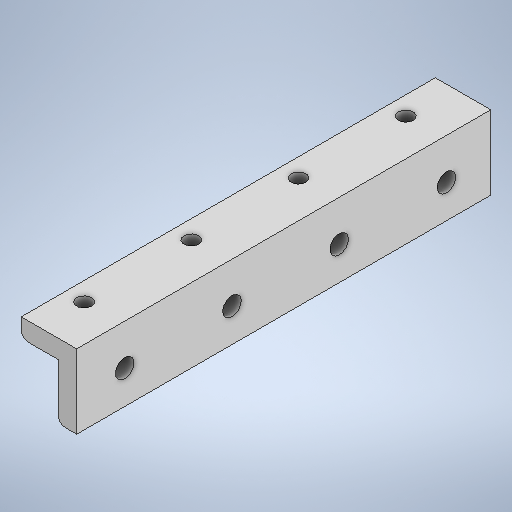
# Autodesk Inventor part: 1014
Saved by Autodesk Inventor 2025.1 (Build 291241000, 241)
## iProperties
Created: 2024-06-10
Part Number: 1014
Material: Generisch
Document SubType Name: Modeling
Designer: ffogue
Density: 1 g/cm^3
Appearance: Vorgabe
Author: ffogue
Autodesk Inventor part; units mm, degrees
ref_plane "YZ Plane" through (0, 0, 0) normal (1, 0, 0) x (0, 1, 0)
ref_plane "XZ Plane" through (0, 0, 0) normal (0, 1, 0) x (-1, 0, 0)
ref_plane "XY Plane" through (0, 0, 0) normal (0, 0, 1) x (1, 0, 0)
sketch "Skizze2" plane through (0, 0, 0) normal (0, 1, 0) x (-1, 0, 0)
  line L0 (0, 0) -> (15, 0)
  line L1 (15, 0) -> (15, -5)
  line L2 (15, -5) -> (5, -5)
  line L3 (5, -5) -> (5, -20)
  line L4 (5, -20) -> (0, -20)
  line L5 (0, -20) -> (0, 0)
  dimension "d6" = 5
  dimension "d7" = 15
  dimension "d8" = 5
  dimension "d9" = 10
  constraints: 12 end point, 5 perpendicular, 1 horizontal
  measures "d6" distance between parallel lines of L2 L0
  measures "d7" distance between parallel lines of L2 L4
  measures "d8" distance between parallel lines of L5 L3
  measures "d9" distance between parallel lines of L3 L1
extrude "Extrusion1" add sketch "Skizze2" along normal blind 112
sketch "Skizze3" plane through (-5, 0, -5) normal (0, 0, -1) x (-1, 0, 0)
  line L0 (0, 112) -> (10, 112) projected
  line L1 (-5, 0) -> (-5, 112) projected
  point P0 (5, 99)
  point P1 (5, 70)
  point P2 (5, 41)
  point P3 (5, 12)
  point P4 (5, 112)
  point P5 (5, 112)
  dimension "d12" = 13
  dimension "d13" = 29
  dimension "d14" = 29
  dimension "d15" = 29
  dimension "d39" = 10
  constraints: 4 vertical alignment, 2 midpoint
  measures "d12" distance of point (5, 112) point (5, 99)
  measures "d13" distance of point (5, 70) point (5, 99)
  measures "d14" distance of point (5, 41) point (5, 70)
  measures "d15" distance of point (5, 12) point (5, 41)
  measures "d39" distance from line of L1 point (5, 99)
hole "Bohrung1" at (-10, 99, -5) at (-10, 70, -5) at (-10, 41, -5) at (-10, 12, -5) direction (0, 0, 1) diameter 4 depth 5 countersink diameter 5 countersink angle 90
sketch "Skizze4" plane through (-5, 0, -20) normal (-1, 0, 0) x (0, 0, 1)
  line L0 (0, 112) -> (15, 112) projected
  line L1 (0, 0) -> (15, 0) projected
  line L2 (20, 0) -> (20, 112) projected
  point P0 (9, 100)
  point P1 (9, 71)
  point P2 (9, 42)
  point P3 (9, 13)
  point P4 (7.5, 0)
  dimension "d30" = 12
  dimension "d31" = 29
  dimension "d32" = 29
  dimension "d33" = 29
  dimension "d40" = 11
  constraints: 3 vertical alignment, 1 midpoint
  measures "d30" distance from line of L0 point (9, 100)
  measures "d31" distance of point (9, 71) point (9, 100)
  measures "d32" distance of point (9, 42) point (9, 71)
  measures "d33" distance of point (9, 13) point (9, 42)
  measures "d40" distance from line of L2 point (9, 13)
hole "Bohrung2" at (-5, 100, -11) at (-5, 71, -11) at (-5, 42, -11) at (-5, 13, -11) direction (1, 0, 0) diameter 5 end through all
fillet "Rundung1" radius 2 2 edges at (-5, 56, -20) (-15, 56, -5)
equation "\"d32\" = d31"
equation "\"d33\" = d32"
